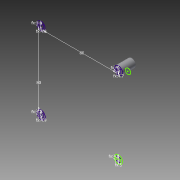
# Autodesk Inventor part: EncoderLDRTube
Saved by Autodesk Inventor 2014 SP1 (Build 180222100, 222)
## iProperties
Created: 2014-07-04
Part Number: EncoderLDRTube
Material: Generic
Document SubType Name: Modeling
Designer: Erin
Density: 1 g/cm^3
Appearance: Default
Author: Erin
Autodesk Inventor part; units mm, degrees
ref_plane "YZ Plane" through (0, 0, 0) normal (1, 0, 0) x (0, 1, 0)
ref_plane "XZ Plane" through (0, 0, 0) normal (0, 1, 0) x (-1, 0, 0)
ref_plane "XY Plane" through (0, 0, 0) normal (0, 0, 1) x (1, 0, 0)
sketch "Sketch1" plane through (0, 0, 0) normal (0, 1, 0) x (-1, 0, 0)
  line L0 (-2.35, 2) -> (2.35, 2)
  line L1 (2.35, 2) -> (2.35, -2)
  line L2 (2.35, -2) -> (-2.35, -2)
  line L3 (-2.35, -2) -> (-2.35, 2)
  circle A0 centre (0, 0) radius 4.5
  line L4 (82.35, 2) -> (87.15, 2)
  line L5 (87.15, 2) -> (87.15, -2.1)
  line L6 (87.15, -2.1) -> (82.35, -2.1)
  line L7 (82.35, -2.1) -> (82.35, 2)
  circle A1 centre (84.75, -0.05) radius 4.5
  line L8 (-2.35, -82.1) -> (2.65, -82.1)
  line L9 (2.65, -82.1) -> (2.65, -86.4)
  line L10 (2.65, -86.4) -> (-2.35, -86.4)
  line L11 (-2.35, -86.4) -> (-2.35, -82.1)
  circle A2 centre (0.15, -84.25) radius 4.5
  line L12 (82.25, -82.1) -> (87.15, -82.1)
  line L13 (87.15, -82.1) -> (87.15, -86.3)
  line L14 (87.15, -86.3) -> (82.25, -86.3)
  line L15 (82.25, -86.3) -> (82.25, -82.1)
  circle A3 centre (84.7, -84.2) radius 4.5
  line L16 (84.75, 2) -> (84.75, -2.1) construction
  line L17 (82.25, -84.2) -> (87.15, -84.2) construction
  line L18 (0.15, -82.1) -> (0.15, -86.4) construction
  circle A4 centre (-10.3312, 4.45) radius 2.9618
  point P0 (0, 2)
  point P1 (2.35, 0)
  point P2 (87.15, -0.05)
  point P3 (2.65, -84.25)
  point P4 (84.7, -82.1)
  dimension "d0" = 4.7
  dimension "d1" = 4
  dimension "d2" = 9
  dimension "d6" = 4.8
  dimension "d7" = 4.1
  dimension "d8" = 9
  dimension "d10" = 5
  dimension "d11" = 4.3
  dimension "d12" = 9
  dimension "d14" = 4.9
  dimension "d15" = 4.2
  dimension "d16" = 9
  dimension "d18" = 80
  dimension "d19" = 80
  constraints: 38 end point, 14 midpoint, 8 parallel, 5 centre point, 5 perpendicular, 4 coincident, 4 horizontal, 3 collinear, 1 horizontal alignment, 1 vertical alignment
  measures "d0" distance of L1.end L2.end
  measures "d1" distance of L0.end L1.end
  measures "d2" diameter of A0
  measures "d6" distance of L5.end L6.end
  measures "d7" distance of L4.end L5.end
  measures "d8" diameter of A1
  measures "d10" distance of L9.end L10.end
  measures "d11" distance of L8.end L9.end
  measures "d12" diameter of A2
  measures "d14" distance of L13.end L14.end
  measures "d15" distance of L12.end L13.end
  measures "d16" diameter of A3
  measures "d18" distance between parallel lines of L7 L1
  measures "d19" distance between parallel lines of L12 L6
extrude "Extrusion1" add sketch "Sketch1" along normal blind 14.5 contours A0
fillet "Fillet1" radius 0.8 4 edges at (-2.35, 7.25, -2) (2.35, 7.25, -2) (2.35, 7.25, 2) (-2.35, 7.25, 2)
extrude "Extrusion2" add sketch "Sketch1" along normal blind 0.6 contours A4
equation "\"sp\" = 0.4"
equation "\"d9\" = 0.4"
equation "\"d13\" = 0.4"
equation "\"d17\" = 0.4"
body "Solid1"
